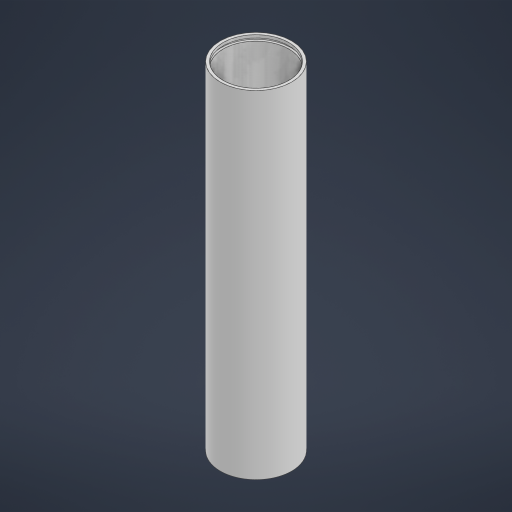
# Autodesk Inventor part: casing
Saved by Autodesk Inventor 2023 (Build 270158000, 158)
## iProperties
Created: 2022-10-07
Part Number: casing
Material: Generic
Document SubType Name: Modeling
Designer: washington
Density: 1 g/cm^3
Appearance: Default
Author: washington
Autodesk Inventor part; units mm, degrees
ref_plane "YZ Plane" through (0, 0, 0) normal (1, 0, 0) x (0, 1, 0)
ref_plane "XZ Plane" through (0, 0, 0) normal (0, 1, 0) x (-1, 0, 0)
ref_plane "XY Plane" through (0, 0, 0) normal (0, 0, 1) x (1, 0, 0)
sketch "Sketch1" plane through (0, 0, 0) normal (0, 1, 0) x (-1, 0, 0)
  circle A0 centre (0, 0) radius 25.4
  circle A1 centre (0, 0) radius 23.4
  dimension "d0" = 50.8
  dimension "d1" = 46.8
  constraints: 2 centre point, 2 coincident
  measures "d0" diameter of A0
  measures "d1" diameter of A1
extrude "Extrusion1" add sketch "Sketch1" along normal mid plane 240
sketch "Sketch2" plane through (0, 0, 0) normal (1, 0, 0) x (0, 1, 0)
  line L0 (120, 23.4) -> (-120, 23.4) projected
  line L1 (118, 23.4) -> (116, 23.4)
  line L2 (116, 23.4) -> (116, 25)
  line L3 (116, 25) -> (118, 25)
  line L4 (118, 25) -> (118, 23.4)
  line L5 (-117, 23.4) -> (-115, 23.4)
  line L6 (-115, 23.4) -> (-115, 25)
  line L7 (-115, 25) -> (-117, 25)
  line L8 (-117, 25) -> (-117, 23.4)
  line L9 (-120, 25.4) -> (-120, -25.4) projected
  line L10 (120, -25.4) -> (120, 25.4) projected
  line L11 (-168, 0) -> (168, 0) projected
  point P0 (0, 0)
  dimension "d4" = 3
  dimension "d5" = 2
  dimension "d6" = 1.6
  dimension "d7" = 2
  dimension "d8" = 2
  dimension "d9" = 1.6
  constraints: 16 end point, 4 parallel, 2 horizontal, 2 perpendicular, 2 point on line
  measures "d4" distance between parallel lines of L9 L8
  measures "d5" distance of L6.end L7.end
  measures "d6" distance between parallel lines of L0 L7
  measures "d7" distance between parallel lines of L10 L4
  measures "d8" distance of L2.end L3.end
  measures "d9" distance between parallel lines of L0 L3
revolve "Revolution1" cut sketch "Sketch2" angle 360 about axis through (0, -10, 0) along (0, 1, 0) contours L0 L2 L3 L4 | L0 L8 L7 L6
body "Solid1"
